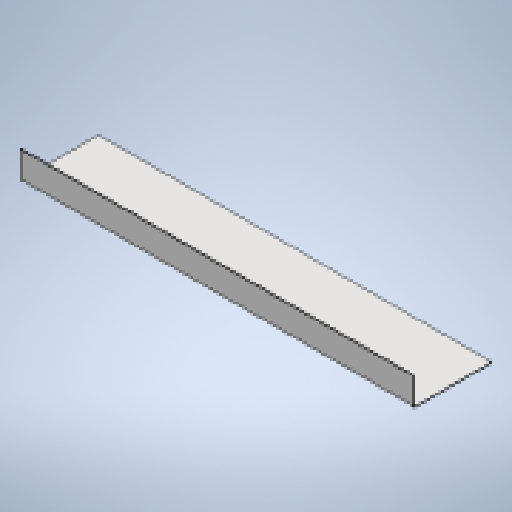
# Autodesk Inventor part: TKS 3006 BOTTOM DS diameter way blind
Saved by Autodesk Inventor 2025.1 (Build 291241020, 241B)
## iProperties
Created: 2024-12-09
Part Number: TKS 3006 BOTTOM DS diameter way blind
Material: Stainless Steel
Document SubType Name: Sheet Metal
Designer: user
Mass: 3269.02 g
Surface Area: 1007.63 cm^2
Volume: 408.627 cm^3
Density: 8 g/cm^3
Flat Pattern Width: 37.3927 cm
Flat Pattern Length: 140 cm
Flat Pattern Area: 5234.98 cm^2
Sheet Metal Rule: AISI304 3mm Die 32
Sheet Metal Width: 373.927 mm
Sheet Metal Length: 1400.000 mm
Sheet Metal Area: 523498.406 mm^2
Appearance: Default
Author: user
Autodesk Inventor part; units mm, degrees
ref_plane "YZ Plane" through (0, 0, 0) normal (1, 0, 0) x (0, 1, 0)
ref_plane "XZ Plane" through (0, 0, 0) normal (0, 1, 0) x (-1, 0, 0)
ref_plane "XY Plane" through (0, 0, 0) normal (0, 0, 1) x (1, 0, 0)
sketch "Sketch1" plane through (0, 0, 0) normal (0, 0, 1) x (1, 0, 0)
  line L0 (700, 140) -> (-700, 140)
  line L1 (-700, 140) -> (-700, -140)
  line L2 (-700, -140) -> (700, -140)
  line L3 (700, -140) -> (700, 140)
  line L4 (700, 140) -> (-700, -140) construction
  line L5 (-700, 140) -> (700, -140) construction
  point P0 (0, 0)
  point P1 (0, 0)
  point P2 (700, 0)
  dimension "d32" = 280
  dimension "d33" = 1400
  measures "d32" distance of L2.end L0.start
  measures "d33" distance of L1.end L2.end
extrude "Plate1" add sketch "Sketch1" along normal blind 3
sketch "Sketch6" plane through (700, -137, 0) normal (0, -1, 0) x (1, 0, 0)
  line L0 (-1400, 0) -> (0, 0)
  line L1 (0, 0) -> (0, 100)
  line L2 (0, 100) -> (-1400, 100)
  line L3 (-1400, 100) -> (-1400, 0)
  constraints: 6 end point, 1 horizontal, 1 perpendicular, 1 vertical
edge flange "Flange2" height 100 angle 90 thickness 3 bend radius 5 thickness toward (0, -1, 0) relief round relief width 3 relief depth 1.5 edges at (0, -140, 3) wall of the first edge with corners at (-700, -137, 0) (700, -137, 0) (700, -137, 100) (-700, -137, 100)
bend "Bend2"
corner "Corner2"
sketch "Sketch8" plane through (0, 0, 3) normal (0, 0, 1) x (1, 0, 0)
  line L0 (646.1751, 51.4978) -> (596.1751, 51.4978)
  line L1 (596.1751, 51.4978) -> (596.1751, 101.4978)
  line L2 (596.1751, 101.4978) -> (646.1751, 101.4978)
  line L3 (646.1751, 101.4978) -> (646.1751, 51.4978)
  line L4 (646.1751, 51.4978) -> (596.1751, 101.4978) construction
  line L5 (596.1751, 51.4978) -> (646.1751, 101.4978) construction
  circle A0 centre (652.9949, 44.678) radius 3.5
  circle A1 centre (589.3553, 44.678) radius 3.5
  circle A2 centre (589.3553, 108.3176) radius 3.5
  circle A3 centre (652.9949, 108.3176) radius 3.5
  circle A4 centre (621.1751, 76.4978) radius 45 construction
  point P0 (0, 0)
  dimension "d51" = 50
  dimension "d52" = 50
  dimension "d53" = 7
  dimension "d54" = 90
  constraints: 12 end point, 5 centre point, 4 point on circle, 4 point on line, 3 equal radius, 2 midpoint, 2 parallel, 1 coincident, 1 horizontal, 1 perpendicular
  measures "d51" distance of L0.start L0.end
  measures "d52" distance of L0.end L1.end
  measures "d53" diameter of A0
  measures "d54" diameter of A4
cut "Cut3" [suppressed]
pattern_linear "Rectangular Pattern1" [suppressed]
equation "\"d55\" = Thickness"
equation "\"d2\" = Thickness"
equation "\"d36\" = BendReliefWidth"
equation "\"d37\" = BendReliefDepth"
equation "\"d38\" = MinimumRemnant"
equation "\"d39\" = TransitionRadius"
equation "\"d42\" = BendRadius"
equation "\"d43\" = CornerReliefSize"
equation "\"d44\" = GapSize"
equation "\"d45\" = JacobiRadiusSize"
equation "\"BendReliefWidth\" = Thickness"
equation "\"BendReliefDepth\" = 0.5 * Thickness"
equation "\"CornerReliefSize\" = 4 * Thickness"
equation "\"MinimumRemnant\" = 2 * Thickness"
equation "\"TransitionRadius\" = BendRadius"
equation "\"JacobiRadiusSize\" = BendRadius"
equation "\"GapSize\" = Thickness"
equation "\"Thickness\" = 3"
equation "\"BendRadius\" = 5"
body "Solid1"
